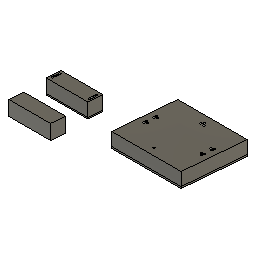
Models (Autodesk Fusion 360 design; units mm, degrees)
Autodesk Fusion 360 part; units mm, degrees
note: some values were not read from the file. Chosen so that the rebuilt part matches the saved one: a direction; where a thread starts. Set by a fixed rule: which sketch regions a step uses.
sketch "Sketch1" plane through (0, 0, 0) normal (0, 0, 1) x (1, 0, 0)
  line L0 (-28.9457, -6.0408) -> (19.0543, -6.0408)
  line L1 (19.0543, -6.0408) -> (20.4541, 9.9592)
  line L2 (20.4541, 9.9592) -> (-27.5459, 9.9592)
  line L3 (-27.5459, 9.9592) -> (-28.9457, -6.0408)
  line L4 (17.6798, -4.5408) -> (18.8172, 8.4592)
  line L5 (18.8172, 8.4592) -> (-26.1714, 8.4592)
  line L6 (-26.1714, 8.4592) -> (-27.3087, -4.5408)
  line L7 (-27.3087, -4.5408) -> (17.6798, -4.5408)
  line L8 (16.5802, -3.3408) -> (17.5076, 7.2592)
  line L9 (-25.0718, 7.2592) -> (-25.9991, -3.3408)
  circle A0 centre (-25.8739, -1.909) radius 1.1
  circle A1 centre (-25.6415, 0.7475) radius 1.1
  circle A2 centre (-25.4091, 3.4041) radius 1.1
  circle A3 centre (16.7055, -1.909) radius 1.1
  line L10 (-24.8394, 9.9158) -> (-25.7667, -0.6842)
  line L11 (-24.6069, 12.5723) -> (-25.5343, 1.9723)
  circle A4 centre (-25.1766, 6.0606) radius 1.1
  line L12 (-24.3745, 15.2288) -> (-25.3019, 4.6288)
  circle A5 centre (16.9379, 0.7475) radius 1.1
  circle A6 centre (17.1703, 3.4041) radius 1.1
  circle A7 centre (17.4027, 6.0606) radius 1.1
  dimension "d1" = 85
  dimension "d2" = 16
  dimension "d3" = 48
  dimension "d4" = -1.5
  dimension "d6" = 2.2
  dimension "d9" = -8
  dimension "d10" = 0
  dimension "d11" = 2.2
  dimension "d14" = 8
  dimension "d15" = 0
  constraint horizontal L0
  constraint parallel L0 L2
  constraint equal L1 L3
  constraint coincident L9 A0.centre
  constraint coincident L8 A3.centre
  measures "d1" angle of L0 L3
  measures "d2" distance of L0 L2
  measures "d3" distance of L1.end L2.end
  measures "d6" diameter of A0
  measures "d11" diameter of A3
extrude "Extrude1" add sketch "Sketch1" against normal blind 15.5 contours L0 L1 L2 L3 makes body 1
extrude "Extrude2" add sketch "Sketch1" against normal blind 2 contours L4 L5 L6 L7 bodies 1
sketch "Sketch2" plane through (0, 0, -15.5) normal (0, 0, -1) x (-1, 0, 0)
  line L0 (27.3087, -4.5408) -> (-17.6798, -4.5408)
  line L1 (26.1714, 8.4592) -> (27.3087, -4.5408)
  line L2 (-18.8172, 8.4592) -> (26.1714, 8.4592)
  line L3 (-17.6798, -4.5408) -> (-18.8172, 8.4592)
  line L4 (28.9457, -6.0408) -> (27.5459, 9.9592)
  line L5 (-19.0543, -6.0408) -> (28.9457, -6.0408)
  line L6 (-20.4541, 9.9592) -> (-19.0543, -6.0408)
  line L7 (27.5459, 9.9592) -> (-20.4541, 9.9592)
extrude "Extrude3" add sketch "Sketch2" against normal blind 1 separate body contours L0 L1 L2 L3 makes body 2
extrude "Extrude4" add 2 faces at (3.4419, 4.1259, -15.5) (-12.4, -5.5408, -15.5) along direction (0, 0, -1) blind 1.5 on bodies 1 2 bodies 2
sketch "Sketch3" plane through (0, 0, 0) normal (0, 0, 1) x (1, 0, 0)
extrude "Extrude5" add sketch "Sketch1" against normal blind 17 separate body contours L0 L1 L2 L3 | L4 L5 L6 L7 | L8 A3 | L8 A3 | L8 A5 | L8 A5 | L8 A6 | L8 A6 | L8 A7 | L8 A7 | L9 L10 L11 A4 L12 | L9 L10 L11 A4 L12 | L9 A2 L10 L11 | L9 A2 L10 L11 | L9 A1 L10 | L9 A1 L10 | L9 A0 | L9 A0 makes body 3
sketch "Sketch4" plane through (0, 0, -17) normal (0, 0, -1) x (1, 0, 0)
  line L0 (-28.9457, 6.0408) -> (-27.5459, -9.9592)
  line L1 (-27.5459, -9.9592) -> (20.4541, -9.9592)
  line L2 (20.4541, -9.9592) -> (19.0543, 6.0408)
  line L3 (19.0543, 6.0408) -> (-28.9457, 6.0408)
  line L4 (-28.2458, -1.9592) -> (19.7542, -1.9592)
  line L5 (-4.2458, 4.3907) -> (-4.2458, -8.7843)
  circle A0 centre (-4.2458, -5.4573) radius 1.825
  circle A1 centre (-4.2458, -5.4573) radius 3.85
  circle A2 centre (-4.2458, 1.5153) radius 3.85
  line L6 (-1.8753, -1.5184) -> (-2.437, -5.7003)
  line L7 (-6.6163, -1.5184) -> (-6.0545, -5.7003)
  line L8 (-8.0958, 1.5153) -> (-8.0958, -5.4573)
  line L9 (-0.3958, -5.4573) -> (-0.3958, 1.5153)
  dimension "d26" = 3.65
  dimension "d27" = 7.7
  dimension "d28" = 7.7
  constraint midpoint L0 L4.start
  constraint midpoint L2 L4.end
  constraint perpendicular L4 L5
  constraint coincident L5 A0.centre
  constraint concentric A0 A1
  constraint coincident L5 A2.centre
  constraint coincident A2 L6.start
  constraint coincident A0 L6.end
  constraint tangent A0 L6
  constraint coincident A2 L7.start
  constraint coincident A0 L7.end
  constraint tangent A0 L7
  constraint coincident A2 L8.start
  constraint coincident A1 L8.end
  constraint tangent A1 L8
  constraint parallel L5 L8
  constraint coincident A1 L9.start
  constraint tangent A1 L9
  constraint parallel L8 L9
  measures "d26" diameter of A0
  measures "d27" diameter of A1
  measures "d28" diameter of A2
extrude "Extrude6" cut sketch "Sketch4" against normal blind 10 contours L4 A2 L7 | L4 A1 A2 L7 | L4 A1 A2 | L4 A1 A2 | L5 A0 A1 A2 L7 | L4 A1 A2 L6 | L4 A2 L6 | L4 L5 A1 | L4 L5 A1 A2 | L5 A0 | L5 A0 A1 A2 L6 | L4 A1 A2 | L4 L5 A1 | L4 L5 A1 A2 | L5 A0 bodies 3
extrude "Extrude7" cut sketch "Sketch4" against normal up to surface (7 mm away) from surface at -3 contours L4 A2 L7 L8 | L4 A1 L7 L8 | A0 A1 L6 L7 | L4 A1 L6 L9 | L4 A2 L6 L9 bodies 3
fillet "Fillet1" radius 3.75 2 edges at (-1.8753, 1.5184, -15.5) (-6.6163, 1.5184, -15.5) on bodies 3
move_body "Move1" bodies 3 to x (1, 0, 0) y (0, 1, 0) z (0, 0, 1) at (0, -43, 0)
sketch "Sketch5" plane through (0, 0, 0) normal (0, 0, 1) x (1, 0, 0)
  line L0 (62.3028, -21.7561) -> (142.3028, -21.7561)
  line L1 (142.3028, -21.7561) -> (148.427, 48.2439)
  line L2 (148.427, 48.2439) -> (68.427, 48.2439)
  line L3 (68.427, 48.2439) -> (62.3028, -21.7561)
  line L4 (140.4701, -19.7561) -> (146.2444, 46.2439)
  line L5 (146.2444, 46.2439) -> (70.2597, 46.2439)
  line L6 (70.2597, 46.2439) -> (64.4854, -19.7561)
  line L7 (64.4854, -19.7561) -> (140.4701, -19.7561)
  line L8 (108.427, 48.2439) -> (102.3028, -21.7561) construction
  circle A0 centre (103, -13.7866) radius 1.1
  circle A1 centre (107.7065, 40.008) radius 1.1
  circle A2 centre (109.475, 37.3075) radius 1.1
  circle A3 centre (105.5065, 37.808) radius 1.1
  line L9 (65.3649, 13.2439) -> (145.3649, 13.2439) construction
  circle A4 centre (72.011, 8.8929) radius 1.1
  circle A5 centre (71.7334, 5.7204) radius 1.1
  circle A6 centre (74.3923, 7.1755) radius 1.1
  line L10 (75.2406, 45.8081) -> (69.4664, -20.1919) construction
  line L11 (72.343, 12.6884) -> (74.6823, 12.4837) construction
  circle A7 centre (72.6751, 16.4839) radius 1.1
  circle A8 centre (75.3185, 17.7617) radius 1.1
  circle A9 centre (72.9527, 19.6564) radius 1.1
  line L12 (105.3649, 13.2439) -> (105.3649, 23.4315) construction
  line L13 (135.4892, -19.3203) -> (141.2634, 46.6797) construction
  circle A10 centre (137.9874, 9.2352) radius 1.1
  circle A11 centre (137.7437, 6.449) radius 1.1
  circle A12 centre (135.4083, 8.2951) radius 1.1
  line L14 (138.3382, 13.2439) -> (133.8944, 13.6327) construction
  circle A13 centre (136.3122, 18.6262) radius 1.1
  circle A14 centre (138.6889, 17.2526) radius 1.1
  circle A15 centre (138.9326, 20.0388) radius 1.1
  dimension "d36" = 85
  dimension "d37" = 70
  dimension "d38" = 80
  dimension "d39" = -2
  dimension "d40" = 2.2
  dimension "d41" = 2.2
  dimension "d42" = 54
  dimension "d43" = 8
  dimension "d44" = 2.2
  dimension "d45" = 2.2
  dimension "d46" = 2.2
  dimension "d47" = 2.2
  dimension "d48" = 2.2
  dimension "d51" = -5
  dimension "d52" = 90
  dimension "d53" = -5
  dimension "d54" = 2.2
  dimension "d55" = 2.2
  dimension "d56" = 2.2
  dimension "d64" = 4
  dimension "d65" = 2.2
  dimension "d66" = 2.2
  constraint horizontal L0
  constraint parallel L0 L2
  constraint equal L1 L3
  constraint midpoint L2 L8.start
  constraint midpoint L0 L8.end
  constraint coincident L8 A0.centre
  constraint coincident L8 A1.centre
  constraint midpoint L3 L9.start
  constraint midpoint L1 L9.end
  constraint coincident A4.centre L10
  constraint coincident A5.centre L10
  constraint coincident L10 L11.start
  constraint symmetric A4 L11 A7
  constraint symmetric A5 L11 A9
  constraint symmetric A6 L11 A8
  constraint midpoint L8 L12.start
  constraint perpendicular L9 L12
  constraint coincident L13 A10.centre
  constraint coincident L13 A11.centre
  constraint coincident L9 L14.start
  constraint coincident L13 L14.start
  constraint perpendicular L13 L14
  constraint symmetric A10 L14 A14
  constraint symmetric A11 L14 A15
  constraint symmetric A12 L14 A13
  measures "d36" angle of L0 L3
  measures "d37" distance of L0 L2
  measures "d38" distance of L0.start L0.end
  measures "d40" diameter of A0
  measures "d41" diameter of A1
  measures "d42" distance of A0.centre A1.centre
  measures "d43" distance of L8.end A0.centre
  measures "d44" diameter of A2
  measures "d45" diameter of A3
  measures "d46" diameter of A4
  measures "d47" diameter of A5
  measures "d48" diameter of A6
  measures "d52" angle of L10 L11
  measures "d54" diameter of A10
  measures "d55" diameter of A11
  measures "d56" diameter of A12
  measures "d64" distance of A2.centre A3.centre
  measures "d65" vertical distance of A1.centre A3.centre
  measures "d66" horizontal distance of A1.centre A3.centre
extrude "Extrude8" add sketch "Sketch5" against normal blind 1.5 separate body contours L0 L1 L2 L3 | L4 L5 L6 L7 makes body 4
extrude "Extrude9" add sketch "Sketch5" against normal blind 15 contours L0 L1 L2 L3 bodies 4
sketch "Sketch6" plane through (0, 0, -1.5) normal (0, 0, -1) x (1, 0, 0)
  line L0 (64.4854, 19.7561) -> (70.2597, -46.2439)
  line L1 (70.2597, -46.2439) -> (146.2444, -46.2439)
  line L2 (146.2444, -46.2439) -> (140.4701, 19.7561)
  line L3 (140.4701, 19.7561) -> (64.4854, 19.7561)
  circle A0 centre (103, 13.7866) radius 1.1
  circle A1 centre (72.6751, -16.4839) radius 1.1
  circle A2 centre (71.7334, -5.7204) radius 1.1
  circle A3 centre (72.9527, -19.6564) radius 1.1
  circle A4 centre (135.4083, -8.2951) radius 1.1
  circle A5 centre (138.9326, -20.0388) radius 1.1
  circle A6 centre (72.011, -8.8929) radius 1.1
  circle A7 centre (137.7437, -6.449) radius 1.1
  circle A8 centre (137.9874, -9.2352) radius 1.1
  circle A9 centre (74.3923, -7.1755) radius 1.1
  circle A10 centre (105.5065, -37.808) radius 1.1
  circle A11 centre (136.3122, -18.6262) radius 1.1
  circle A12 centre (107.7065, -40.008) radius 1.1
  circle A13 centre (109.475, -37.3075) radius 1.1
  circle A14 centre (138.6889, -17.2526) radius 1.1
  circle A15 centre (75.3185, -17.7617) radius 1.1
  line L4 (64.4854, 19.7561) -> (146.2444, -46.2439) construction
  line L5 (70.2597, -46.2439) -> (140.4701, 19.7561) construction
  circle A16 centre (105.3649, -13.2439) radius 1.5
  circle A17 centre (105.3649, -13.2439) radius 4
  dimension "d67" = 3
  dimension "d68" = 8
  constraint coincident L0.start L3.end
  constraint coincident L1.end L2.start
  constraint coincident L0.end L1.start
  constraint coincident L2.end L3.start
  constraint midpoint L4 A16.centre
  constraint concentric A16 A17
  measures "d67" diameter of A16
  measures "d68" diameter of A17
extrude "Extrude10" add sketch "Sketch6" along normal up to surface (13.5 mm away) contours A17 bodies 4
thread "Thread1" "ISO Metric profile 3.0 M3x0.5 M3x0.5 6H" major diameter 3.086 minor diameter 2.529 pitch 0.5 angle 60 modelled right hand crest width 0.1368 on face at (106.514, 12.2797, -10.5) crest through (106.6294, 13.2439, -14.625) on bodies 4
chamfer "Chamfer1" distance 3 distance2 5.5 1 edges at (101.6356, 11.7974, -1.5) measured on face at (127.1912, -9.239, -1.5) on bodies 4
chamfer "Chamfer2" distance 0.5 angle 45 1 edges at (101.6356, 11.7974, -15) on bodies 4
fillet "Fillet2" radius 2.25 2 edges at (98.8386, 15.7752, -1.5) (101.6356, 11.7974, -7) on bodies 4
sketch "Sketch7" plane through (0, 0, -15) normal (0, 0, -1) x (1, 0, 0)
  line L0 (64.4854, 19.7561) -> (140.4701, 19.7561)
  line L1 (140.4701, 19.7561) -> (146.2444, -46.2439)
  line L2 (146.2444, -46.2439) -> (70.2597, -46.2439)
  line L3 (70.2597, -46.2439) -> (64.4854, 19.7561)
  line L4 (62.3028, 21.7561) -> (68.427, -48.2439)
  line L5 (68.427, -48.2439) -> (148.427, -48.2439)
  line L6 (148.427, -48.2439) -> (142.3028, 21.7561)
  line L7 (142.3028, 21.7561) -> (62.3028, 21.7561)
  spline S0 degree 3 poles (105.7634, -11.7532) (105.9483, -11.8208) (106.1184, -11.9232) (106.4038, -12.1837) (106.5181, -12.3374) (106.6773, -12.6743) (106.723, -12.8531) (106.7416, -13.2113) (106.7169, -13.3871) (106.6239, -13.652) (106.5774, -13.7467) (106.4639, -13.9204) (106.3979, -13.9992) (106.323, -14.0691) knots 0 0 0 0 0.059039 0.059039 0.116033 0.116033 0.170983 0.170983 0.223888 0.223888 0.255505 0.255505 0.286347 0.286347 0.286347 0.286347
  arc A0 (104.4068, -14.0691) -> (106.323, -14.0691) centre (105.3649, -13.2439) ccw
  spline S1 degree 3 poles (104.4068, -14.0691) (104.2847, -13.9551) (104.1865, -13.8179) (104.0442, -13.5079) (104.0038, -13.3369) (103.9892, -12.9821) (104.0178, -12.8016) (104.1437, -12.4548) (104.2423, -12.2926) (104.4493, -12.0647) (104.5405, -11.9862) (104.7417, -11.851) (104.8513, -11.7953) (104.9664, -11.7532) knots 0 0 0 0 0.050111 0.050111 0.102261 0.102261 0.15645 0.15645 0.212677 0.212677 0.24852 0.24852 0.285143 0.285143 0.285143 0.285143
  arc A1 (105.7634, -11.7532) -> (104.9664, -11.7532) centre (105.3649, -13.2439) ccw
  circle A2 centre (105.3649, -13.2439) radius 3.5
  circle A3 centre (105.3649, -13.2439) radius 1.6
  circle A4 centre (105.3649, -13.2439) radius 4.5
  dimension "d78" = 3.2
  dimension "d79" = 9
  constraint concentric A0 A3
  constraint concentric A3 A4
  measures "d78" diameter of A3
  measures "d79" diameter of A4
extrude "Extrude11" add sketch "Sketch7" against normal blind 0.5 separate body contours L0 L1 L2 L3 makes body 5
extrude "Extrude12" add 2 faces at (78.5367, 13.2439, -15) (89.697, -21.0894, -15) along direction (0, 0, -1) blind 2 on bodies 4 5 bodies 5
extrude "Extrude13" add sketch "Sketch7" along normal blind 2 contours A2 | A4 bodies 5
chamfer "Chamfer3" distance 2.5 distance2 2 1 edges at (103.8732, 12.6653, -17) measured on face at (78.1649, 13.2439, -17) on bodies 5
delete_face "DeleteFace1" [no effect]
delete_face "DeleteFace2" [no effect]
sketch "Sketch8" plane through (0, 0, -1.5) normal (0, 0, -1) x (1, 0, 0)
  circle A0 centre (138.9326, -20.0388) radius 1.1
  circle A1 centre (105.5065, -37.808) radius 1.1
  circle A2 centre (137.9874, -9.2352) radius 1.1
  circle A3 centre (74.3923, -7.1755) radius 1.1
  circle A4 centre (75.3185, -17.7617) radius 1.1
  circle A5 centre (109.475, -37.3075) radius 1.1
  circle A6 centre (135.4083, -8.2951) radius 1.1
  circle A7 centre (72.9527, -19.6564) radius 1.1
  circle A8 centre (72.011, -8.8929) radius 1.1
  circle A9 centre (107.7065, -40.008) radius 1.1
  circle A10 centre (103, 13.7866) radius 1.1
  circle A11 centre (137.7437, -6.449) radius 1.1
  circle A12 centre (71.7334, -5.7204) radius 1.1
  circle A13 centre (136.3122, -18.6262) radius 1.1
  circle A14 centre (72.6751, -16.4839) radius 1.1
  circle A15 centre (138.6889, -17.2526) radius 1.1
  line L0 (64.4854, 19.7561) -> (70.2597, -46.2439)
  line L1 (70.2597, -46.2439) -> (146.2444, -46.2439)
  line L2 (146.2444, -46.2439) -> (140.4701, 19.7561)
  line L3 (140.4701, 19.7561) -> (64.4854, 19.7561)
  circle A16 centre (105.3649, -13.2439) radius 8.3357
equation "d38 = ( 16 * 5 ) * 1 mm"
equation "d43 = ( 70 mm - d42 ) / 2"
equation "d51 = d53"
equation "d66 = d65"
